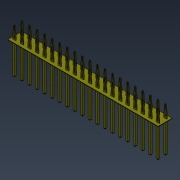
# Autodesk Inventor part: ESQ-120-33-T-D_pins
Saved by Autodesk Inventor 2022.1 (Build 261234020, 234B)
## iProperties
Created: 2017-11-11
Part Number: ESQ-120-33-T-D_pins
Catalog Web Link: www.cadenas.de
Description: ESQ Series Pins-ESQ Series - (2,54 mm) .100'' Elevated Socket
Vendor: SAMTEC
Document SubType Name: Modeling
Designer: psAdmin
Manufacturer: SAMTEC
Mass: 0.221213 g
Surface Area: 18.7913 cm^2
Volume: 0.221213 cm^3
Density: 1 g/cm^3
Material: Allgemein
Appearance: PSOLRGB-255-255-0
Category: PARTsolutions
Company: SAMTEC
PSOL_IDENT_0: {$CADENAS_DATA\23d-libs\samtec\modelling\esq\parts\esq_pins.prj},218 {VTYP=3D},{NB=ESQ-120-33-T-D_pi
PSOL_IDENT_1: ns},{LINA=ESQ-120-33-T-D_pins},{NN=ESQ Series Pins},{DATE=21.05.2015 12:04:42},{GEOMDATE=21.05.2015
PSOL_IDENT_2: 12:04:00},{VERSION=},{LINEID=10},{LINESUBID=-1},{WBVAR=POS,LS,PLOPT,ROW,LLOPT,POLOPT}  {NB=ESQ-120-3
PSOL_IDENT_3: 3-T-D_pins},{LINA=ESQ-120-33-T-D_pins},{KT=DUMMY},{PN=ESQ-120-33-T-D},{SERIES=ESQ},{POS=20},{POSN=20
PSOL_IDENT_4: },{POSALG=  '01','-01','02','-02','03','-03','04','-04','05','-05','06','-06','07','-07','08','-08','
PSOL_IDENT_5: 09','-09','10','-10','11','-11','12','-12','13','-13','14','-14','15','-15','16','-16','17','-17','1
PSOL_IDENT_6: 8','-18','19','-19','20','-20','21','-21','22','-22','23','-23','24','-24','25','-25','26','-26','27'
PSOL_IDENT_7: ,'-27','28','-28','29','-29','30','-30','31','-31','32','-32','33','-33','34','-34','35','-35','36','
PSOL_IDENT_8: -36'  },{POSPN=20},{LS=33},{PLOPT=T},{PLOPTALG= 'G','-G = 20micro\" Selective Gold in Contact Area,
PSOL_IDENT_9: 3micro\" Selective Gold on Tail.','T','-T = Matte Tin on Entire Pin.','S','-S =  30micro\" Selective
PSOL_IDENT_10: Gold in Contact Area, Matte Tin on Tail.','H','-H = 30micro\" Selective Gold in Contact Area, 3micr
PSOL_IDENT_11: o\" Selective Gold on Tail.','F','-F = 3micro\" Selective Gold in Contact Area, Matte Tin on Tail.','
PSOL_IDENT_12: E','-E = 50micro\" Selective Gold in Contact Area, 3micro\" Selective Gold on Tail.','L','-L = 10mic
PSOL_IDENT_13: ro\" Selective Gold in Contact Area, Matte Tin on Tail.' },{ROW=D},{ROWPN=-D},{ROWALG= 'S','-S = Sin
PSOL_IDENT_14: gle Row','D','-D = Double Row','T','-T = Triple Row' },{ROWN=2},{LLOPT=},{LLOPTALG= '','Not Selected'
PSOL_IDENT_15: ,'LL','-LL = Locking Lead' },{LLOPTPN=},{POLOPT=},{POLOPTPN=},{POLOPTMAX=480},{POLOPTMAX2='001','001'
PSOL_IDENT_16: ,'002','002','003','003','004','004','005','005','006','006','007','007','008','008','009','009','01
PSOL_IDENT_17: 0','010','011','011','012','012','013','013','014','014','015','015','016','016','017','017','018','
PSOL_IDENT_18: 018','019','019','020','020','021','021','022','022','023','023','024','024','025','025','026','026'
PSOL_IDENT_19: ,'027','027','028','028','029','029','030','030','031','031','032','032','033','033','034','034','03
PSOL_IDENT_20: 5','035','036','036','037','037','038','038','039','039','040','040'},{POLOPTALG= '','Not Selected','
PSOL_IDENT_21: 001','001','002','002','003','003','004','004','005','005','006','006','007','007','008','008','009'
PSOL_IDENT_22: ,'009','010','010','011','011','012','012','013','013','014','014','015','015','016','016','017','01
PSOL_IDENT_23: 7','018','018','019','019','020','020','021','021','022','022','023','023','024','024','025','025','
PSOL_IDENT_24: 026','026','027','027','028','028','029','029','030','030','031','031','032','032','033','033','034'
PSOL_IDENT_25: ,'034','035','035','036','036','037','037','038','038','039','039','040','040'},{POLARIZE='001','001'
PSOL_IDENT_26: ,'002','002','003','003','004','004','005','005','006','006','007','007','008','008','009','009','01
PSOL_IDENT_27: 0','010','011','011','012','012','013','013','014','014','015','015','016','016','017','017','018','
PSOL_IDENT_28: 018','019','019','020','020','021','021','022','022','023','023','024','024','025','025','026','026'
PSOL_IDENT_29: ,'027','027','028','028','029','029','030','030','031','031','032','032','033','033','034','034','03
PSOL_IDENT_30: 5','035','036','036','037','037','038','038','039','039','040','040','041','041','042','042','043','
PSOL_IDENT_31: 043','044','044','045','045','046','046','047','047','048','048','049','049','050','050','051','051'
PSOL_IDENT_32: ,'052','052','053','053','054','054','055','055','056','056','057','057','058','058','059','059','06
PSOL_IDENT_33: 0','060','061','061','062','062','063','063','064','064','065','065','066','066','067','067','068','
PSOL_IDENT_34: 068','069','069','070','070','071','071','072','072','073','073','074','074','075','075','076','076'
PSOL_IDENT_35: ,'077','077','078','078','079','079','080','080','081','081','082','082','083','083','084','084','08
PSOL_IDENT_36: 5','085','086','086','087','087','088','088','089','089','090','090','091','091','092','092','093','
PSOL_IDENT_37: 093','094','094','095','095','096','096','097','097','098','098','099','099','100','100','101','101'
PSOL_IDENT_38: ,'102','102','103','103','104','104','105','105','106','106','107','107','108','108','109','109','11
PSOL_IDENT_39: 0','110','111','111','112','112','113','113','114','114','115','115','116','116','117','117','118','
PSOL_IDENT_40: 118','119','119','120','120','121','121','122','122','123','123','124','124','125','125','126','126'
PSOL_IDENT_41: ,'127','127','128','128','129','129','130','130','131','131','132','132','133','133','134','134','13
PSOL_IDENT_42: 5','135','136','136','137','137','138','138','139','139','140','140','141','141','142','142','143','
PSOL_IDENT_43: 143','144','144','145','145','146','146','147','147','148','148','149','149','150','150','151','151'
PSOL_IDENT_44: ,'152','152','153','153','154','154','155','155','156','156','157','157','158','158','159','159','16
PSOL_IDENT_45: 0','160','161','161','162','162','163','163','164','164','165','165','166','166','167','167','168','
PSOL_IDENT_46: 168','169','169','170','170','171','171','172','172','173','173','174','174','175','175','176','176'
PSOL_IDENT_47: ,'177','177','178','178','179','179','180','180','181','181','182','182','183','183','184','184','18
PSOL_IDENT_48: 5','185','186','186','187','187','188','188','189','189','190','190','191','191','192','192','193','
PSOL_IDENT_49: 193','194','194','195','195','196','196','197','197','198','198','199','199','200','200','201','201'
PSOL_IDENT_50: ,'202','202','203','203','204','204','205','205','206','206','207','207','208','208','209','209','21
PSOL_IDENT_51: 0','210','211','211','212','212','213','213','214','214','215','215','216','216','217','217','218','
PSOL_IDENT_52: 218','219','219','220','220','221','221','222','222','223','223','224','224','225','225','226','226'
PSOL_IDENT_53: ,'227','227','228','228','229','229','230','230','231','231','232','232','233','233','234','234','23
PSOL_IDENT_54: 5','235','236','236','237','237','238','238','239','239','240','240','241','241','242','242','243','
PSOL_IDENT_55: 243','244','244','245','245','246','246','247','247','248','248','249','249','250','250','251','251'
PSOL_IDENT_56: ,'252','252','253','253','254','254','255','255','256','256','257','257','258','258','259','259','26
PSOL_IDENT_57: 0','260','261','261','262','262','263','263','264','264','265','265','266','266','267','267','268','
PSOL_IDENT_58: 268','269','269','270','270','271','271','272','272','273','273','274','274','275','275','276','276'
PSOL_IDENT_59: ,'277','277','278','278','279','279','280','280','281','281','282','282','283','283','284','284','28
PSOL_IDENT_60: 5','285','286','286','287','287','288','288','289','289','290','290','291','291','292','292','293','
PSOL_IDENT_61: 293','294','294','295','295','296','296','297','297','298','298','299','299','300','300'},{POLARIZEX=
PSOL_IDENT_62: 0.00000},{POLARIZEY=0.00000},{POLARIZEN=0},{EVEN=0},{EVENLL=1},{A=0.195},{A3DB=0.33500},{B=0.09000},
PSOL_IDENT_63: {C=0.635},{D=0.725},{E=0.000},{W=2.02000}
NN: ESQ Series Pins
NT: ESQ Series - (2,54 mm) .100'' Elevated Socket
NB: ESQ-120-33-T-D_pins
NBSYN: $PN._pins
LINA: ESQ-120-33-T-D_pins
PN: ESQ-120-33-T-D
SERIES: ESQ
POS: -20
LS: -33
PLOPT: -T = Matte Tin on Entire Pin.
ROW: -D = Double Row
LLOPT: Not Selected
POLOPT: Not Selected
A: 0.195
W: 2.02000
SUPPLIER: SAMTEC
ARTICLENO: ESQ-120-33-T-D_pins
BOMINFO: ESQ-120-33-T-D_pins
CREATOR: CADENAS GmbH
Title: ESQ-120-33-T-D_pins
Author: Cadenas PARTsolutions
Comments: ESQ Series - (2,54 mm) .100'' Elevated Socket
Autodesk Inventor part; units mm, degrees
sketch "Sketch_1" plane through (0, -9.906, 0) normal (0, 1, 0) x (1, 0, 0)
  line L0 (-25.273, 2.3495) -> (-25.273, -2.3495)
  line L1 (-25.273, -2.3495) -> (25.273, -2.3495)
  line L2 (25.273, -2.3495) -> (25.273, 2.3495)
  line L3 (25.273, 2.3495) -> (-25.273, 2.3495)
  constraints: 8 end point
extrude "Extrusion1" add sketch "Sketch_1" along normal blind 15.494
sketch "Sketch_2" plane through (0, 0.635, 0) normal (0, 1, 0) x (1, 0, 0)
  line L0 (-25.654, 2.4765) -> (-25.654, -2.4765)
  line L1 (-25.654, -2.4765) -> (25.654, -2.4765)
  line L2 (25.654, -2.4765) -> (25.654, 2.4765)
  line L3 (25.654, 2.4765) -> (-25.654, 2.4765)
  line L4 (23.8125, -0.9525) -> (23.8125, -1.5875)
  line L5 (23.8125, -1.5875) -> (24.4475, -1.5875)
  line L6 (24.4475, -1.5875) -> (24.4475, -0.9525)
  line L7 (24.4475, -0.9525) -> (23.8125, -0.9525)
  line L8 (23.8125, 1.5875) -> (23.8125, 0.9525)
  line L9 (23.8125, 0.9525) -> (24.4475, 0.9525)
  line L10 (24.4475, 0.9525) -> (24.4475, 1.5875)
  line L11 (24.4475, 1.5875) -> (23.8125, 1.5875)
  line L12 (21.2725, -0.9525) -> (21.2725, -1.5875)
  line L13 (21.2725, -1.5875) -> (21.9075, -1.5875)
  line L14 (21.9075, -1.5875) -> (21.9075, -0.9525)
  line L15 (21.9075, -0.9525) -> (21.2725, -0.9525)
  line L16 (21.2725, 1.5875) -> (21.2725, 0.9525)
  line L17 (21.2725, 0.9525) -> (21.9075, 0.9525)
  line L18 (21.9075, 0.9525) -> (21.9075, 1.5875)
  line L19 (21.9075, 1.5875) -> (21.2725, 1.5875)
  line L20 (18.7325, -0.9525) -> (18.7325, -1.5875)
  line L21 (18.7325, -1.5875) -> (19.3675, -1.5875)
  line L22 (19.3675, -1.5875) -> (19.3675, -0.9525)
  line L23 (19.3675, -0.9525) -> (18.7325, -0.9525)
  line L24 (18.7325, 1.5875) -> (18.7325, 0.9525)
  line L25 (18.7325, 0.9525) -> (19.3675, 0.9525)
  line L26 (19.3675, 0.9525) -> (19.3675, 1.5875)
  line L27 (19.3675, 1.5875) -> (18.7325, 1.5875)
  line L28 (16.1925, -0.9525) -> (16.1925, -1.5875)
  line L29 (16.1925, -1.5875) -> (16.8275, -1.5875)
  line L30 (16.8275, -1.5875) -> (16.8275, -0.9525)
  line L31 (16.8275, -0.9525) -> (16.1925, -0.9525)
  line L32 (16.1925, 1.5875) -> (16.1925, 0.9525)
  line L33 (16.1925, 0.9525) -> (16.8275, 0.9525)
  line L34 (16.8275, 0.9525) -> (16.8275, 1.5875)
  line L35 (16.8275, 1.5875) -> (16.1925, 1.5875)
  line L36 (13.6525, -0.9525) -> (13.6525, -1.5875)
  line L37 (13.6525, -1.5875) -> (14.2875, -1.5875)
  line L38 (14.2875, -1.5875) -> (14.2875, -0.9525)
  line L39 (14.2875, -0.9525) -> (13.6525, -0.9525)
  line L40 (13.6525, 1.5875) -> (13.6525, 0.9525)
  line L41 (13.6525, 0.9525) -> (14.2875, 0.9525)
  line L42 (14.2875, 0.9525) -> (14.2875, 1.5875)
  line L43 (14.2875, 1.5875) -> (13.6525, 1.5875)
  line L44 (11.1125, -0.9525) -> (11.1125, -1.5875)
  line L45 (11.1125, -1.5875) -> (11.7475, -1.5875)
  line L46 (11.7475, -1.5875) -> (11.7475, -0.9525)
  line L47 (11.7475, -0.9525) -> (11.1125, -0.9525)
  line L48 (11.1125, 1.5875) -> (11.1125, 0.9525)
  line L49 (11.1125, 0.9525) -> (11.7475, 0.9525)
  line L50 (11.7475, 0.9525) -> (11.7475, 1.5875)
  line L51 (11.7475, 1.5875) -> (11.1125, 1.5875)
  line L52 (8.5725, -0.9525) -> (8.5725, -1.5875)
  line L53 (8.5725, -1.5875) -> (9.2075, -1.5875)
  line L54 (9.2075, -1.5875) -> (9.2075, -0.9525)
  line L55 (9.2075, -0.9525) -> (8.5725, -0.9525)
  line L56 (8.5725, 1.5875) -> (8.5725, 0.9525)
  line L57 (8.5725, 0.9525) -> (9.2075, 0.9525)
  line L58 (9.2075, 0.9525) -> (9.2075, 1.5875)
  line L59 (9.2075, 1.5875) -> (8.5725, 1.5875)
  line L60 (6.0325, -0.9525) -> (6.0325, -1.5875)
  line L61 (6.0325, -1.5875) -> (6.6675, -1.5875)
  line L62 (6.6675, -1.5875) -> (6.6675, -0.9525)
  line L63 (6.6675, -0.9525) -> (6.0325, -0.9525)
  line L64 (6.0325, 1.5875) -> (6.0325, 0.9525)
  line L65 (6.0325, 0.9525) -> (6.6675, 0.9525)
  line L66 (6.6675, 0.9525) -> (6.6675, 1.5875)
  line L67 (6.6675, 1.5875) -> (6.0325, 1.5875)
  line L68 (3.4925, -0.9525) -> (3.4925, -1.5875)
  line L69 (3.4925, -1.5875) -> (4.1275, -1.5875)
  line L70 (4.1275, -1.5875) -> (4.1275, -0.9525)
  line L71 (4.1275, -0.9525) -> (3.4925, -0.9525)
  line L72 (3.4925, 1.5875) -> (3.4925, 0.9525)
  line L73 (3.4925, 0.9525) -> (4.1275, 0.9525)
  line L74 (4.1275, 0.9525) -> (4.1275, 1.5875)
  line L75 (4.1275, 1.5875) -> (3.4925, 1.5875)
  line L76 (0.9525, -0.9525) -> (0.9525, -1.5875)
  line L77 (0.9525, -1.5875) -> (1.5875, -1.5875)
  line L78 (1.5875, -1.5875) -> (1.5875, -0.9525)
  line L79 (1.5875, -0.9525) -> (0.9525, -0.9525)
  line L80 (0.9525, 1.5875) -> (0.9525, 0.9525)
  line L81 (0.9525, 0.9525) -> (1.5875, 0.9525)
  line L82 (1.5875, 0.9525) -> (1.5875, 1.5875)
  line L83 (1.5875, 1.5875) -> (0.9525, 1.5875)
  line L84 (-1.5875, -0.9525) -> (-1.5875, -1.5875)
  line L85 (-1.5875, -1.5875) -> (-0.9525, -1.5875)
  line L86 (-0.9525, -1.5875) -> (-0.9525, -0.9525)
  line L87 (-0.9525, -0.9525) -> (-1.5875, -0.9525)
  line L88 (-1.5875, 1.5875) -> (-1.5875, 0.9525)
  line L89 (-1.5875, 0.9525) -> (-0.9525, 0.9525)
  line L90 (-0.9525, 0.9525) -> (-0.9525, 1.5875)
  line L91 (-0.9525, 1.5875) -> (-1.5875, 1.5875)
  line L92 (-4.1275, -0.9525) -> (-4.1275, -1.5875)
  line L93 (-4.1275, -1.5875) -> (-3.4925, -1.5875)
  line L94 (-3.4925, -1.5875) -> (-3.4925, -0.9525)
  line L95 (-3.4925, -0.9525) -> (-4.1275, -0.9525)
  line L96 (-4.1275, 1.5875) -> (-4.1275, 0.9525)
  line L97 (-4.1275, 0.9525) -> (-3.4925, 0.9525)
  line L98 (-3.4925, 0.9525) -> (-3.4925, 1.5875)
  line L99 (-3.4925, 1.5875) -> (-4.1275, 1.5875)
  line L100 (-6.6675, -0.9525) -> (-6.6675, -1.5875)
  line L101 (-6.6675, -1.5875) -> (-6.0325, -1.5875)
  line L102 (-6.0325, -1.5875) -> (-6.0325, -0.9525)
  line L103 (-6.0325, -0.9525) -> (-6.6675, -0.9525)
  line L104 (-6.6675, 1.5875) -> (-6.6675, 0.9525)
  line L105 (-6.6675, 0.9525) -> (-6.0325, 0.9525)
  line L106 (-6.0325, 0.9525) -> (-6.0325, 1.5875)
  line L107 (-6.0325, 1.5875) -> (-6.6675, 1.5875)
  line L108 (-9.2075, -0.9525) -> (-9.2075, -1.5875)
  line L109 (-9.2075, -1.5875) -> (-8.5725, -1.5875)
  line L110 (-8.5725, -1.5875) -> (-8.5725, -0.9525)
  line L111 (-8.5725, -0.9525) -> (-9.2075, -0.9525)
  line L112 (-9.2075, 1.5875) -> (-9.2075, 0.9525)
  line L113 (-9.2075, 0.9525) -> (-8.5725, 0.9525)
  line L114 (-8.5725, 0.9525) -> (-8.5725, 1.5875)
  line L115 (-8.5725, 1.5875) -> (-9.2075, 1.5875)
  line L116 (-11.7475, -0.9525) -> (-11.7475, -1.5875)
  line L117 (-11.7475, -1.5875) -> (-11.1125, -1.5875)
  line L118 (-11.1125, -1.5875) -> (-11.1125, -0.9525)
  line L119 (-11.1125, -0.9525) -> (-11.7475, -0.9525)
  line L120 (-11.7475, 1.5875) -> (-11.7475, 0.9525)
  line L121 (-11.7475, 0.9525) -> (-11.1125, 0.9525)
  line L122 (-11.1125, 0.9525) -> (-11.1125, 1.5875)
  line L123 (-11.1125, 1.5875) -> (-11.7475, 1.5875)
  line L124 (-14.2875, -0.9525) -> (-14.2875, -1.5875)
  line L125 (-14.2875, -1.5875) -> (-13.6525, -1.5875)
  line L126 (-13.6525, -1.5875) -> (-13.6525, -0.9525)
  line L127 (-13.6525, -0.9525) -> (-14.2875, -0.9525)
  line L128 (-14.2875, 1.5875) -> (-14.2875, 0.9525)
  line L129 (-14.2875, 0.9525) -> (-13.6525, 0.9525)
  line L130 (-13.6525, 0.9525) -> (-13.6525, 1.5875)
  line L131 (-13.6525, 1.5875) -> (-14.2875, 1.5875)
  line L132 (-16.8275, -0.9525) -> (-16.8275, -1.5875)
  line L133 (-16.8275, -1.5875) -> (-16.1925, -1.5875)
  line L134 (-16.1925, -1.5875) -> (-16.1925, -0.9525)
  line L135 (-16.1925, -0.9525) -> (-16.8275, -0.9525)
  line L136 (-16.8275, 1.5875) -> (-16.8275, 0.9525)
  line L137 (-16.8275, 0.9525) -> (-16.1925, 0.9525)
  line L138 (-16.1925, 0.9525) -> (-16.1925, 1.5875)
  line L139 (-16.1925, 1.5875) -> (-16.8275, 1.5875)
  line L140 (-19.3675, -0.9525) -> (-19.3675, -1.5875)
  line L141 (-19.3675, -1.5875) -> (-18.7325, -1.5875)
  line L142 (-18.7325, -1.5875) -> (-18.7325, -0.9525)
  line L143 (-18.7325, -0.9525) -> (-19.3675, -0.9525)
  line L144 (-19.3675, 1.5875) -> (-19.3675, 0.9525)
  line L145 (-19.3675, 0.9525) -> (-18.7325, 0.9525)
  line L146 (-18.7325, 0.9525) -> (-18.7325, 1.5875)
  line L147 (-18.7325, 1.5875) -> (-19.3675, 1.5875)
  line L148 (-21.9075, -0.9525) -> (-21.9075, -1.5875)
  line L149 (-21.9075, -1.5875) -> (-21.2725, -1.5875)
  line L150 (-21.2725, -1.5875) -> (-21.2725, -0.9525)
  line L151 (-21.2725, -0.9525) -> (-21.9075, -0.9525)
  line L152 (-21.9075, 1.5875) -> (-21.9075, 0.9525)
  line L153 (-21.9075, 0.9525) -> (-21.2725, 0.9525)
  line L154 (-21.2725, 0.9525) -> (-21.2725, 1.5875)
  line L155 (-21.2725, 1.5875) -> (-21.9075, 1.5875)
  line L156 (-24.4475, -0.9525) -> (-24.4475, -1.5875)
  line L157 (-24.4475, -1.5875) -> (-23.8125, -1.5875)
  line L158 (-23.8125, -1.5875) -> (-23.8125, -0.9525)
  line L159 (-23.8125, -0.9525) -> (-24.4475, -0.9525)
  line L160 (-24.4475, 1.5875) -> (-24.4475, 0.9525)
  line L161 (-24.4475, 0.9525) -> (-23.8125, 0.9525)
  line L162 (-23.8125, 0.9525) -> (-23.8125, 1.5875)
  line L163 (-23.8125, 1.5875) -> (-24.4475, 1.5875)
  constraints: 328 end point
extrude "Extrusion2" cut sketch "Sketch_2" against normal blind 10.668
sketch "Sketch_4" plane through (0, 0, 0) normal (1, 0, 0) x (0, 1, 0)
  line L0 (-10.414, 3.81) -> (-11.684, 3.81)
  line L1 (-11.684, 3.81) -> (-11.684, -3.4925)
  line L2 (-11.684, -3.4925) -> (-10.414, -3.4925)
  line L3 (-10.414, -3.4925) -> (-10.414, -1.5875)
  line L4 (-10.414, -1.5875) -> (-9.652, -1.5875)
  line L5 (-9.652, -1.5875) -> (-10.2019, -1.27)
  line L6 (-10.2019, -1.27) -> (-9.652, -0.9525)
  line L7 (-9.652, -0.9525) -> (-10.414, -0.9525)
  line L8 (-10.414, -0.9525) -> (-10.414, 0.9525)
  line L9 (-10.414, 0.9525) -> (-9.652, 0.9525)
  line L10 (-9.652, 0.9525) -> (-10.2019, 1.27)
  line L11 (-10.2019, 1.27) -> (-9.652, 1.5875)
  line L12 (-9.652, 1.5875) -> (-10.414, 1.5875)
  line L13 (-10.414, 1.5875) -> (-10.414, 3.81)
  constraints: 28 end point
extrude "Extrusion3" cut sketch "Sketch_4" along normal mid plane 102.616
sketch "Sketch_7" plane through (0, 0, 0) normal (0, 0, 1) x (1, 0, 0)
  line L0 (-25.4, -10.922) -> (-25.4, -12.192)
  line L1 (-25.4, -12.192) -> (26.3525, -12.192)
  line L2 (26.3525, -12.192) -> (26.3525, -10.922)
  line L3 (26.3525, -10.922) -> (24.4475, -10.922)
  line L4 (24.4475, -10.922) -> (24.4475, -9.652)
  line L5 (24.4475, -9.652) -> (24.13, -10.2019)
  line L6 (24.13, -10.2019) -> (23.8125, -9.652)
  line L7 (23.8125, -9.652) -> (23.8125, -10.922)
  line L8 (23.8125, -10.922) -> (21.9075, -10.922)
  line L9 (21.9075, -10.922) -> (21.9075, -9.652)
  line L10 (21.9075, -9.652) -> (21.59, -10.2019)
  line L11 (21.59, -10.2019) -> (21.2725, -9.652)
  line L12 (21.2725, -9.652) -> (21.2725, -10.922)
  line L13 (21.2725, -10.922) -> (19.3675, -10.922)
  line L14 (19.3675, -10.922) -> (19.3675, -9.652)
  line L15 (19.3675, -9.652) -> (19.05, -10.2019)
  line L16 (19.05, -10.2019) -> (18.7325, -9.652)
  line L17 (18.7325, -9.652) -> (18.7325, -10.922)
  line L18 (18.7325, -10.922) -> (16.8275, -10.922)
  line L19 (16.8275, -10.922) -> (16.8275, -9.652)
  line L20 (16.8275, -9.652) -> (16.51, -10.2019)
  line L21 (16.51, -10.2019) -> (16.1925, -9.652)
  line L22 (16.1925, -9.652) -> (16.1925, -10.922)
  line L23 (16.1925, -10.922) -> (14.2875, -10.922)
  line L24 (14.2875, -10.922) -> (14.2875, -9.652)
  line L25 (14.2875, -9.652) -> (13.97, -10.2019)
  line L26 (13.97, -10.2019) -> (13.6525, -9.652)
  line L27 (13.6525, -9.652) -> (13.6525, -10.922)
  line L28 (13.6525, -10.922) -> (11.7475, -10.922)
  line L29 (11.7475, -10.922) -> (11.7475, -9.652)
  line L30 (11.7475, -9.652) -> (11.43, -10.2019)
  line L31 (11.43, -10.2019) -> (11.1125, -9.652)
  line L32 (11.1125, -9.652) -> (11.1125, -10.922)
  line L33 (11.1125, -10.922) -> (9.2075, -10.922)
  line L34 (9.2075, -10.922) -> (9.2075, -9.652)
  line L35 (9.2075, -9.652) -> (8.89, -10.2019)
  line L36 (8.89, -10.2019) -> (8.5725, -9.652)
  line L37 (8.5725, -9.652) -> (8.5725, -10.922)
  line L38 (8.5725, -10.922) -> (6.6675, -10.922)
  line L39 (6.6675, -10.922) -> (6.6675, -9.652)
  line L40 (6.6675, -9.652) -> (6.35, -10.2019)
  line L41 (6.35, -10.2019) -> (6.0325, -9.652)
  line L42 (6.0325, -9.652) -> (6.0325, -10.922)
  line L43 (6.0325, -10.922) -> (4.1275, -10.922)
  line L44 (4.1275, -10.922) -> (4.1275, -9.652)
  line L45 (4.1275, -9.652) -> (3.81, -10.2019)
  line L46 (3.81, -10.2019) -> (3.4925, -9.652)
  line L47 (3.4925, -9.652) -> (3.4925, -10.922)
  line L48 (3.4925, -10.922) -> (1.5875, -10.922)
  line L49 (1.5875, -10.922) -> (1.5875, -9.652)
  line L50 (1.5875, -9.652) -> (1.27, -10.2019)
  line L51 (1.27, -10.2019) -> (0.9525, -9.652)
  line L52 (0.9525, -9.652) -> (0.9525, -10.922)
  line L53 (0.9525, -10.922) -> (-0.9525, -10.922)
  line L54 (-0.9525, -10.922) -> (-0.9525, -9.652)
  line L55 (-0.9525, -9.652) -> (-1.27, -10.2019)
  line L56 (-1.27, -10.2019) -> (-1.5875, -9.652)
  line L57 (-1.5875, -9.652) -> (-1.5875, -10.922)
  line L58 (-1.5875, -10.922) -> (-3.4925, -10.922)
  line L59 (-3.4925, -10.922) -> (-3.4925, -9.652)
  line L60 (-3.4925, -9.652) -> (-3.81, -10.2019)
  line L61 (-3.81, -10.2019) -> (-4.1275, -9.652)
  line L62 (-4.1275, -9.652) -> (-4.1275, -10.922)
  line L63 (-4.1275, -10.922) -> (-6.0325, -10.922)
  line L64 (-6.0325, -10.922) -> (-6.0325, -9.652)
  line L65 (-6.0325, -9.652) -> (-6.35, -10.2019)
  line L66 (-6.35, -10.2019) -> (-6.6675, -9.652)
  line L67 (-6.6675, -9.652) -> (-6.6675, -10.922)
  line L68 (-6.6675, -10.922) -> (-8.5725, -10.922)
  line L69 (-8.5725, -10.922) -> (-8.5725, -9.652)
  line L70 (-8.5725, -9.652) -> (-8.89, -10.2019)
  line L71 (-8.89, -10.2019) -> (-9.2075, -9.652)
  line L72 (-9.2075, -9.652) -> (-9.2075, -10.922)
  line L73 (-9.2075, -10.922) -> (-11.1125, -10.922)
  line L74 (-11.1125, -10.922) -> (-11.1125, -9.652)
  line L75 (-11.1125, -9.652) -> (-11.43, -10.2019)
  line L76 (-11.43, -10.2019) -> (-11.7475, -9.652)
  line L77 (-11.7475, -9.652) -> (-11.7475, -10.922)
  line L78 (-11.7475, -10.922) -> (-13.6525, -10.922)
  line L79 (-13.6525, -10.922) -> (-13.6525, -9.652)
  line L80 (-13.6525, -9.652) -> (-13.97, -10.2019)
  line L81 (-13.97, -10.2019) -> (-14.2875, -9.652)
  line L82 (-14.2875, -9.652) -> (-14.2875, -10.922)
  line L83 (-14.2875, -10.922) -> (-16.1925, -10.922)
  line L84 (-16.1925, -10.922) -> (-16.1925, -9.652)
  line L85 (-16.1925, -9.652) -> (-16.51, -10.2019)
  line L86 (-16.51, -10.2019) -> (-16.8275, -9.652)
  line L87 (-16.8275, -9.652) -> (-16.8275, -10.922)
  line L88 (-16.8275, -10.922) -> (-18.7325, -10.922)
  line L89 (-18.7325, -10.922) -> (-18.7325, -9.652)
  line L90 (-18.7325, -9.652) -> (-19.05, -10.2019)
  line L91 (-19.05, -10.2019) -> (-19.3675, -9.652)
  line L92 (-19.3675, -9.652) -> (-19.3675, -10.922)
  line L93 (-19.3675, -10.922) -> (-21.2725, -10.922)
  line L94 (-21.2725, -10.922) -> (-21.2725, -9.652)
  line L95 (-21.2725, -9.652) -> (-21.59, -10.2019)
  line L96 (-21.59, -10.2019) -> (-21.9075, -9.652)
  line L97 (-21.9075, -9.652) -> (-21.9075, -10.922)
  line L98 (-21.9075, -10.922) -> (-23.8125, -10.922)
  line L99 (-23.8125, -10.922) -> (-23.8125, -9.652)
  line L100 (-23.8125, -9.652) -> (-24.13, -10.2019)
  line L101 (-24.13, -10.2019) -> (-24.4475, -9.652)
  line L102 (-24.4475, -9.652) -> (-24.4475, -10.922)
  line L103 (-24.4475, -10.922) -> (-25.4, -10.922)
  constraints: 208 end point
extrude "Extrusion4" cut sketch "Sketch_7" along normal mid plane 9.906
sketch "Sketch_10" plane through (0, 0.762, 0) normal (0, 1, 0) x (1, 0, 0)
  line L0 (-25.654, 2.4765) -> (-25.654, -2.4765)
  line L1 (-25.654, -2.4765) -> (25.654, -2.4765)
  line L2 (25.654, -2.4765) -> (25.654, 2.4765)
  line L3 (25.654, 2.4765) -> (-25.654, 2.4765)
  line L4 (23.622, -1.143) -> (23.622, -1.397)
  line L5 (23.622, -1.397) -> (24.638, -1.397)
  line L6 (24.638, -1.397) -> (24.638, -1.143)
  line L7 (24.638, -1.143) -> (23.622, -1.143)
  line L8 (23.622, 1.397) -> (23.622, 1.143)
  line L9 (23.622, 1.143) -> (24.638, 1.143)
  line L10 (24.638, 1.143) -> (24.638, 1.397)
  line L11 (24.638, 1.397) -> (23.622, 1.397)
  line L12 (21.082, -1.143) -> (21.082, -1.397)
  line L13 (21.082, -1.397) -> (22.098, -1.397)
  line L14 (22.098, -1.397) -> (22.098, -1.143)
  line L15 (22.098, -1.143) -> (21.082, -1.143)
  line L16 (21.082, 1.397) -> (21.082, 1.143)
  line L17 (21.082, 1.143) -> (22.098, 1.143)
  line L18 (22.098, 1.143) -> (22.098, 1.397)
  line L19 (22.098, 1.397) -> (21.082, 1.397)
  line L20 (18.542, -1.143) -> (18.542, -1.397)
  line L21 (18.542, -1.397) -> (19.558, -1.397)
  line L22 (19.558, -1.397) -> (19.558, -1.143)
  line L23 (19.558, -1.143) -> (18.542, -1.143)
  line L24 (18.542, 1.397) -> (18.542, 1.143)
  line L25 (18.542, 1.143) -> (19.558, 1.143)
  line L26 (19.558, 1.143) -> (19.558, 1.397)
  line L27 (19.558, 1.397) -> (18.542, 1.397)
  line L28 (16.002, -1.143) -> (16.002, -1.397)
  line L29 (16.002, -1.397) -> (17.018, -1.397)
  line L30 (17.018, -1.397) -> (17.018, -1.143)
  line L31 (17.018, -1.143) -> (16.002, -1.143)
  line L32 (16.002, 1.397) -> (16.002, 1.143)
  line L33 (16.002, 1.143) -> (17.018, 1.143)
  line L34 (17.018, 1.143) -> (17.018, 1.397)
  line L35 (17.018, 1.397) -> (16.002, 1.397)
  line L36 (13.462, -1.143) -> (13.462, -1.397)
  line L37 (13.462, -1.397) -> (14.478, -1.397)
  line L38 (14.478, -1.397) -> (14.478, -1.143)
  line L39 (14.478, -1.143) -> (13.462, -1.143)
  line L40 (13.462, 1.397) -> (13.462, 1.143)
  line L41 (13.462, 1.143) -> (14.478, 1.143)
  line L42 (14.478, 1.143) -> (14.478, 1.397)
  line L43 (14.478, 1.397) -> (13.462, 1.397)
  line L44 (10.922, -1.143) -> (10.922, -1.397)
  line L45 (10.922, -1.397) -> (11.938, -1.397)
  line L46 (11.938, -1.397) -> (11.938, -1.143)
  line L47 (11.938, -1.143) -> (10.922, -1.143)
  line L48 (10.922, 1.397) -> (10.922, 1.143)
  line L49 (10.922, 1.143) -> (11.938, 1.143)
  line L50 (11.938, 1.143) -> (11.938, 1.397)
  line L51 (11.938, 1.397) -> (10.922, 1.397)
  line L52 (8.382, -1.143) -> (8.382, -1.397)
  line L53 (8.382, -1.397) -> (9.398, -1.397)
  line L54 (9.398, -1.397) -> (9.398, -1.143)
  line L55 (9.398, -1.143) -> (8.382, -1.143)
  line L56 (8.382, 1.397) -> (8.382, 1.143)
  line L57 (8.382, 1.143) -> (9.398, 1.143)
  line L58 (9.398, 1.143) -> (9.398, 1.397)
  line L59 (9.398, 1.397) -> (8.382, 1.397)
  line L60 (5.842, -1.143) -> (5.842, -1.397)
  line L61 (5.842, -1.397) -> (6.858, -1.397)
  line L62 (6.858, -1.397) -> (6.858, -1.143)
  line L63 (6.858, -1.143) -> (5.842, -1.143)
  line L64 (5.842, 1.397) -> (5.842, 1.143)
  line L65 (5.842, 1.143) -> (6.858, 1.143)
  line L66 (6.858, 1.143) -> (6.858, 1.397)
  line L67 (6.858, 1.397) -> (5.842, 1.397)
  line L68 (3.302, -1.143) -> (3.302, -1.397)
  line L69 (3.302, -1.397) -> (4.318, -1.397)
  line L70 (4.318, -1.397) -> (4.318, -1.143)
  line L71 (4.318, -1.143) -> (3.302, -1.143)
  line L72 (3.302, 1.397) -> (3.302, 1.143)
  line L73 (3.302, 1.143) -> (4.318, 1.143)
  line L74 (4.318, 1.143) -> (4.318, 1.397)
  line L75 (4.318, 1.397) -> (3.302, 1.397)
  line L76 (0.762, -1.143) -> (0.762, -1.397)
  line L77 (0.762, -1.397) -> (1.778, -1.397)
  line L78 (1.778, -1.397) -> (1.778, -1.143)
  line L79 (1.778, -1.143) -> (0.762, -1.143)
  line L80 (0.762, 1.397) -> (0.762, 1.143)
  line L81 (0.762, 1.143) -> (1.778, 1.143)
  line L82 (1.778, 1.143) -> (1.778, 1.397)
  line L83 (1.778, 1.397) -> (0.762, 1.397)
  line L84 (-1.778, -1.143) -> (-1.778, -1.397)
  line L85 (-1.778, -1.397) -> (-0.762, -1.397)
  line L86 (-0.762, -1.397) -> (-0.762, -1.143)
  line L87 (-0.762, -1.143) -> (-1.778, -1.143)
  line L88 (-1.778, 1.397) -> (-1.778, 1.143)
  line L89 (-1.778, 1.143) -> (-0.762, 1.143)
  line L90 (-0.762, 1.143) -> (-0.762, 1.397)
  line L91 (-0.762, 1.397) -> (-1.778, 1.397)
  line L92 (-4.318, -1.143) -> (-4.318, -1.397)
  line L93 (-4.318, -1.397) -> (-3.302, -1.397)
  line L94 (-3.302, -1.397) -> (-3.302, -1.143)
  line L95 (-3.302, -1.143) -> (-4.318, -1.143)
  line L96 (-4.318, 1.397) -> (-4.318, 1.143)
  line L97 (-4.318, 1.143) -> (-3.302, 1.143)
  line L98 (-3.302, 1.143) -> (-3.302, 1.397)
  line L99 (-3.302, 1.397) -> (-4.318, 1.397)
  line L100 (-6.858, -1.143) -> (-6.858, -1.397)
  line L101 (-6.858, -1.397) -> (-5.842, -1.397)
  line L102 (-5.842, -1.397) -> (-5.842, -1.143)
  line L103 (-5.842, -1.143) -> (-6.858, -1.143)
  line L104 (-6.858, 1.397) -> (-6.858, 1.143)
  line L105 (-6.858, 1.143) -> (-5.842, 1.143)
  line L106 (-5.842, 1.143) -> (-5.842, 1.397)
  line L107 (-5.842, 1.397) -> (-6.858, 1.397)
  line L108 (-9.398, -1.143) -> (-9.398, -1.397)
  line L109 (-9.398, -1.397) -> (-8.382, -1.397)
  line L110 (-8.382, -1.397) -> (-8.382, -1.143)
  line L111 (-8.382, -1.143) -> (-9.398, -1.143)
  line L112 (-9.398, 1.397) -> (-9.398, 1.143)
  line L113 (-9.398, 1.143) -> (-8.382, 1.143)
  line L114 (-8.382, 1.143) -> (-8.382, 1.397)
  line L115 (-8.382, 1.397) -> (-9.398, 1.397)
  line L116 (-11.938, -1.143) -> (-11.938, -1.397)
  line L117 (-11.938, -1.397) -> (-10.922, -1.397)
  line L118 (-10.922, -1.397) -> (-10.922, -1.143)
  line L119 (-10.922, -1.143) -> (-11.938, -1.143)
  line L120 (-11.938, 1.397) -> (-11.938, 1.143)
  line L121 (-11.938, 1.143) -> (-10.922, 1.143)
  line L122 (-10.922, 1.143) -> (-10.922, 1.397)
  line L123 (-10.922, 1.397) -> (-11.938, 1.397)
  line L124 (-14.478, -1.143) -> (-14.478, -1.397)
  line L125 (-14.478, -1.397) -> (-13.462, -1.397)
  line L126 (-13.462, -1.397) -> (-13.462, -1.143)
  line L127 (-13.462, -1.143) -> (-14.478, -1.143)
  line L128 (-14.478, 1.397) -> (-14.478, 1.143)
  line L129 (-14.478, 1.143) -> (-13.462, 1.143)
  line L130 (-13.462, 1.143) -> (-13.462, 1.397)
  line L131 (-13.462, 1.397) -> (-14.478, 1.397)
  line L132 (-17.018, -1.143) -> (-17.018, -1.397)
  line L133 (-17.018, -1.397) -> (-16.002, -1.397)
  line L134 (-16.002, -1.397) -> (-16.002, -1.143)
  line L135 (-16.002, -1.143) -> (-17.018, -1.143)
  line L136 (-17.018, 1.397) -> (-17.018, 1.143)
  line L137 (-17.018, 1.143) -> (-16.002, 1.143)
  line L138 (-16.002, 1.143) -> (-16.002, 1.397)
  line L139 (-16.002, 1.397) -> (-17.018, 1.397)
  line L140 (-19.558, -1.143) -> (-19.558, -1.397)
  line L141 (-19.558, -1.397) -> (-18.542, -1.397)
  line L142 (-18.542, -1.397) -> (-18.542, -1.143)
  line L143 (-18.542, -1.143) -> (-19.558, -1.143)
  line L144 (-19.558, 1.397) -> (-19.558, 1.143)
  line L145 (-19.558, 1.143) -> (-18.542, 1.143)
  line L146 (-18.542, 1.143) -> (-18.542, 1.397)
  line L147 (-18.542, 1.397) -> (-19.558, 1.397)
  line L148 (-22.098, -1.143) -> (-22.098, -1.397)
  line L149 (-22.098, -1.397) -> (-21.082, -1.397)
  line L150 (-21.082, -1.397) -> (-21.082, -1.143)
  line L151 (-21.082, -1.143) -> (-22.098, -1.143)
  line L152 (-22.098, 1.397) -> (-22.098, 1.143)
  line L153 (-22.098, 1.143) -> (-21.082, 1.143)
  line L154 (-21.082, 1.143) -> (-21.082, 1.397)
  line L155 (-21.082, 1.397) -> (-22.098, 1.397)
  line L156 (-24.638, -1.143) -> (-24.638, -1.397)
  line L157 (-24.638, -1.397) -> (-23.622, -1.397)
  line L158 (-23.622, -1.397) -> (-23.622, -1.143)
  line L159 (-23.622, -1.143) -> (-24.638, -1.143)
  line L160 (-24.638, 1.397) -> (-24.638, 1.143)
  line L161 (-24.638, 1.143) -> (-23.622, 1.143)
  line L162 (-23.622, 1.143) -> (-23.622, 1.397)
  line L163 (-23.622, 1.397) -> (-24.638, 1.397)
  constraints: 328 end point
extrude "Extrusion5" cut sketch "Sketch_10" along normal blind 4.826
sketch "Sketch_12" plane through (0, 0, 0) normal (0, 0, 1) x (1, 0, 0)
  line L0 (-25.654, 8.9535) -> (-25.654, 1.3335)
  line L1 (-25.654, 1.3335) -> (-24.6662, 1.3335)
  line L2 (-24.6662, 1.3335) -> (-24.2951, 4.9444)
  line L3 (-24.2951, 4.9444) -> (-24.1681, 4.7244)
  line L4 (-24.1681, 4.7244) -> (-24.3203, 1.3421)
  arc A0 (-24.3203, 1.3421) -> (-23.9397, 1.3421) centre (-24.13, 1.3335) ccw
  line L5 (-23.9397, 1.3421) -> (-24.0919, 4.7244)
  line L6 (-24.0919, 4.7244) -> (-23.9649, 4.9444)
  line L7 (-23.9649, 4.9444) -> (-23.5938, 1.3335)
  line L8 (-23.5938, 1.3335) -> (-22.1262, 1.3335)
  line L9 (-22.1262, 1.3335) -> (-21.7551, 4.9444)
  line L10 (-21.7551, 4.9444) -> (-21.6281, 4.7244)
  line L11 (-21.6281, 4.7244) -> (-21.7803, 1.3421)
  arc A1 (-21.7803, 1.3421) -> (-21.3997, 1.3421) centre (-21.59, 1.3335) ccw
  line L12 (-21.3997, 1.3421) -> (-21.5519, 4.7244)
  line L13 (-21.5519, 4.7244) -> (-21.4249, 4.9444)
  line L14 (-21.4249, 4.9444) -> (-21.0538, 1.3335)
  line L15 (-21.0538, 1.3335) -> (-19.5862, 1.3335)
  line L16 (-19.5862, 1.3335) -> (-19.2151, 4.9444)
  line L17 (-19.2151, 4.9444) -> (-19.0881, 4.7244)
  line L18 (-19.0881, 4.7244) -> (-19.2403, 1.3421)
  arc A2 (-19.2403, 1.3421) -> (-18.8597, 1.3421) centre (-19.05, 1.3335) ccw
  line L19 (-18.8597, 1.3421) -> (-19.0119, 4.7244)
  line L20 (-19.0119, 4.7244) -> (-18.8849, 4.9444)
  line L21 (-18.8849, 4.9444) -> (-18.5138, 1.3335)
  line L22 (-18.5138, 1.3335) -> (-17.0462, 1.3335)
  line L23 (-17.0462, 1.3335) -> (-16.6751, 4.9444)
  line L24 (-16.6751, 4.9444) -> (-16.5481, 4.7244)
  line L25 (-16.5481, 4.7244) -> (-16.7003, 1.3421)
  arc A3 (-16.7003, 1.3421) -> (-16.3197, 1.3421) centre (-16.51, 1.3335) ccw
  line L26 (-16.3197, 1.3421) -> (-16.4719, 4.7244)
  line L27 (-16.4719, 4.7244) -> (-16.3449, 4.9444)
  line L28 (-16.3449, 4.9444) -> (-15.9738, 1.3335)
  line L29 (-15.9738, 1.3335) -> (-14.5062, 1.3335)
  line L30 (-14.5062, 1.3335) -> (-14.1351, 4.9444)
  line L31 (-14.1351, 4.9444) -> (-14.0081, 4.7244)
  line L32 (-14.0081, 4.7244) -> (-14.1603, 1.3421)
  arc A4 (-14.1603, 1.3421) -> (-13.7797, 1.3421) centre (-13.97, 1.3335) ccw
  line L33 (-13.7797, 1.3421) -> (-13.9319, 4.7244)
  line L34 (-13.9319, 4.7244) -> (-13.8049, 4.9444)
  line L35 (-13.8049, 4.9444) -> (-13.4338, 1.3335)
  line L36 (-13.4338, 1.3335) -> (-11.9662, 1.3335)
  line L37 (-11.9662, 1.3335) -> (-11.5951, 4.9444)
  line L38 (-11.5951, 4.9444) -> (-11.4681, 4.7244)
  line L39 (-11.4681, 4.7244) -> (-11.6203, 1.3421)
  arc A5 (-11.6203, 1.3421) -> (-11.2397, 1.3421) centre (-11.43, 1.3335) ccw
  line L40 (-11.2397, 1.3421) -> (-11.3919, 4.7244)
  line L41 (-11.3919, 4.7244) -> (-11.2649, 4.9444)
  line L42 (-11.2649, 4.9444) -> (-10.8938, 1.3335)
  line L43 (-10.8938, 1.3335) -> (-9.4262, 1.3335)
  line L44 (-9.4262, 1.3335) -> (-9.0551, 4.9444)
  line L45 (-9.0551, 4.9444) -> (-8.9281, 4.7244)
  line L46 (-8.9281, 4.7244) -> (-9.0803, 1.3421)
  arc A6 (-9.0803, 1.3421) -> (-8.6997, 1.3421) centre (-8.89, 1.3335) ccw
  line L47 (-8.6997, 1.3421) -> (-8.8519, 4.7244)
  line L48 (-8.8519, 4.7244) -> (-8.7249, 4.9444)
  line L49 (-8.7249, 4.9444) -> (-8.3538, 1.3335)
  line L50 (-8.3538, 1.3335) -> (-6.8862, 1.3335)
  line L51 (-6.8862, 1.3335) -> (-6.5151, 4.9444)
  line L52 (-6.5151, 4.9444) -> (-6.3881, 4.7244)
  line L53 (-6.3881, 4.7244) -> (-6.5403, 1.3421)
  arc A7 (-6.5403, 1.3421) -> (-6.1597, 1.3421) centre (-6.35, 1.3335) ccw
  line L54 (-6.1597, 1.3421) -> (-6.3119, 4.7244)
  line L55 (-6.3119, 4.7244) -> (-6.1849, 4.9444)
  line L56 (-6.1849, 4.9444) -> (-5.8138, 1.3335)
  line L57 (-5.8138, 1.3335) -> (-4.3462, 1.3335)
  line L58 (-4.3462, 1.3335) -> (-3.9751, 4.9444)
  line L59 (-3.9751, 4.9444) -> (-3.8481, 4.7244)
  line L60 (-3.8481, 4.7244) -> (-4.0003, 1.3421)
  arc A8 (-4.0003, 1.3421) -> (-3.6197, 1.3421) centre (-3.81, 1.3335) ccw
  line L61 (-3.6197, 1.3421) -> (-3.7719, 4.7244)
  line L62 (-3.7719, 4.7244) -> (-3.6449, 4.9444)
  line L63 (-3.6449, 4.9444) -> (-3.2738, 1.3335)
  line L64 (-3.2738, 1.3335) -> (-1.8062, 1.3335)
  line L65 (-1.8062, 1.3335) -> (-1.4351, 4.9444)
  line L66 (-1.4351, 4.9444) -> (-1.3081, 4.7244)
  line L67 (-1.3081, 4.7244) -> (-1.4603, 1.3421)
  arc A9 (-1.4603, 1.3421) -> (-1.0797, 1.3421) centre (-1.27, 1.3335) ccw
  line L68 (-1.0797, 1.3421) -> (-1.2319, 4.7244)
  line L69 (-1.2319, 4.7244) -> (-1.1049, 4.9444)
  line L70 (-1.1049, 4.9444) -> (-0.7338, 1.3335)
  line L71 (-0.7338, 1.3335) -> (0.7338, 1.3335)
  line L72 (0.7338, 1.3335) -> (1.1049, 4.9444)
  line L73 (1.1049, 4.9444) -> (1.2319, 4.7244)
  line L74 (1.2319, 4.7244) -> (1.0797, 1.3421)
  arc A10 (1.0797, 1.3421) -> (1.4603, 1.3421) centre (1.27, 1.3335) ccw
  line L75 (1.4603, 1.3421) -> (1.3081, 4.7244)
  line L76 (1.3081, 4.7244) -> (1.4351, 4.9444)
  line L77 (1.4351, 4.9444) -> (1.8062, 1.3335)
  line L78 (1.8062, 1.3335) -> (3.2738, 1.3335)
  line L79 (3.2738, 1.3335) -> (3.6449, 4.9444)
  line L80 (3.6449, 4.9444) -> (3.7719, 4.7244)
  line L81 (3.7719, 4.7244) -> (3.6197, 1.3421)
  arc A11 (3.6197, 1.3421) -> (4.0003, 1.3421) centre (3.81, 1.3335) ccw
  line L82 (4.0003, 1.3421) -> (3.8481, 4.7244)
  line L83 (3.8481, 4.7244) -> (3.9751, 4.9444)
  line L84 (3.9751, 4.9444) -> (4.3462, 1.3335)
  line L85 (4.3462, 1.3335) -> (5.8138, 1.3335)
  line L86 (5.8138, 1.3335) -> (6.1849, 4.9444)
  line L87 (6.1849, 4.9444) -> (6.3119, 4.7244)
  line L88 (6.3119, 4.7244) -> (6.1597, 1.3421)
  arc A12 (6.1597, 1.3421) -> (6.5403, 1.3421) centre (6.35, 1.3335) ccw
  line L89 (6.5403, 1.3421) -> (6.3881, 4.7244)
  line L90 (6.3881, 4.7244) -> (6.5151, 4.9444)
  line L91 (6.5151, 4.9444) -> (6.8862, 1.3335)
  line L92 (6.8862, 1.3335) -> (8.3538, 1.3335)
  line L93 (8.3538, 1.3335) -> (8.7249, 4.9444)
  line L94 (8.7249, 4.9444) -> (8.8519, 4.7244)
  line L95 (8.8519, 4.7244) -> (8.6997, 1.3421)
  arc A13 (8.6997, 1.3421) -> (9.0803, 1.3421) centre (8.89, 1.3335) ccw
  line L96 (9.0803, 1.3421) -> (8.9281, 4.7244)
  line L97 (8.9281, 4.7244) -> (9.0551, 4.9444)
  line L98 (9.0551, 4.9444) -> (9.4262, 1.3335)
  line L99 (9.4262, 1.3335) -> (10.8938, 1.3335)
  line L100 (10.8938, 1.3335) -> (11.2649, 4.9444)
  line L101 (11.2649, 4.9444) -> (11.3919, 4.7244)
  line L102 (11.3919, 4.7244) -> (11.2397, 1.3421)
  arc A14 (11.2397, 1.3421) -> (11.6203, 1.3421) centre (11.43, 1.3335) ccw
  line L103 (11.6203, 1.3421) -> (11.4681, 4.7244)
  line L104 (11.4681, 4.7244) -> (11.5951, 4.9444)
  line L105 (11.5951, 4.9444) -> (11.9662, 1.3335)
  line L106 (11.9662, 1.3335) -> (13.4338, 1.3335)
  line L107 (13.4338, 1.3335) -> (13.8049, 4.9444)
  line L108 (13.8049, 4.9444) -> (13.9319, 4.7244)
  line L109 (13.9319, 4.7244) -> (13.7797, 1.3421)
  arc A15 (13.7797, 1.3421) -> (14.1603, 1.3421) centre (13.97, 1.3335) ccw
  line L110 (14.1603, 1.3421) -> (14.0081, 4.7244)
  line L111 (14.0081, 4.7244) -> (14.1351, 4.9444)
  line L112 (14.1351, 4.9444) -> (14.5062, 1.3335)
  line L113 (14.5062, 1.3335) -> (15.9738, 1.3335)
  line L114 (15.9738, 1.3335) -> (16.3449, 4.9444)
  line L115 (16.3449, 4.9444) -> (16.4719, 4.7244)
  line L116 (16.4719, 4.7244) -> (16.3197, 1.3421)
  arc A16 (16.3197, 1.3421) -> (16.7003, 1.3421) centre (16.51, 1.3335) ccw
  line L117 (16.7003, 1.3421) -> (16.5481, 4.7244)
  line L118 (16.5481, 4.7244) -> (16.6751, 4.9444)
  line L119 (16.6751, 4.9444) -> (17.0462, 1.3335)
  line L120 (17.0462, 1.3335) -> (18.5138, 1.3335)
  line L121 (18.5138, 1.3335) -> (18.8849, 4.9444)
  line L122 (18.8849, 4.9444) -> (19.0119, 4.7244)
  line L123 (19.0119, 4.7244) -> (18.8597, 1.3421)
  arc A17 (18.8597, 1.3421) -> (19.2403, 1.3421) centre (19.05, 1.3335) ccw
  line L124 (19.2403, 1.3421) -> (19.0881, 4.7244)
  line L125 (19.0881, 4.7244) -> (19.2151, 4.9444)
  line L126 (19.2151, 4.9444) -> (19.5862, 1.3335)
  line L127 (19.5862, 1.3335) -> (21.0538, 1.3335)
  line L128 (21.0538, 1.3335) -> (21.4249, 4.9444)
  line L129 (21.4249, 4.9444) -> (21.5519, 4.7244)
  line L130 (21.5519, 4.7244) -> (21.3997, 1.3421)
  arc A18 (21.3997, 1.3421) -> (21.7803, 1.3421) centre (21.59, 1.3335) ccw
  line L131 (21.7803, 1.3421) -> (21.6281, 4.7244)
  line L132 (21.6281, 4.7244) -> (21.7551, 4.9444)
  line L133 (21.7551, 4.9444) -> (22.1262, 1.3335)
  line L134 (22.1262, 1.3335) -> (23.5938, 1.3335)
  line L135 (23.5938, 1.3335) -> (23.9649, 4.9444)
  line L136 (23.9649, 4.9444) -> (24.0919, 4.7244)
  line L137 (24.0919, 4.7244) -> (23.9397, 1.3421)
  arc A19 (23.9397, 1.3421) -> (24.3203, 1.3421) centre (24.13, 1.3335) ccw
  line L138 (24.3203, 1.3421) -> (24.1681, 4.7244)
  line L139 (24.1681, 4.7244) -> (24.2951, 4.9444)
  line L140 (24.2951, 4.9444) -> (24.6662, 1.3335)
  line L141 (24.6662, 1.3335) -> (26.1493, 1.3335)
  line L142 (26.1493, 1.3335) -> (26.1493, 8.9535)
  line L143 (26.1493, 8.9535) -> (-25.654, 8.9535)
  constraints: 288 end point, 40 point on circle, 20 centre point
extrude "Extrusion6" cut sketch "Sketch_12" along normal mid plane 9.906
ref_plane "pins_XY" through (0, 0, 0) normal (0, 1, 0) x (1, 0, 0)
ref_plane "pins_YZ" through (0, 0, 0) normal (1, 0, 0) x (0, 0, -1)
ref_plane "pins_ZX" through (0, 0, 0) normal (0, 0, -1) x (0, 1, 0)
body "Solid1"
